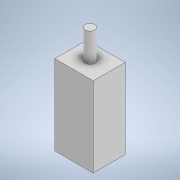
# Autodesk Inventor part: мотор_для_шестерни
Saved by Autodesk Inventor 2021.1 (Build 251245010, 245A)
## iProperties
Created: 2022-04-01
Part Number: мотор_для_шестерни
Material: Типовые
Document SubType Name: Modeling
Designer: zmoze
Density: 1 g/cm^3
Appearance: По умолчанию
Author: zmoze
Autodesk Inventor part; units mm, degrees
ref_plane "YZ Plane" through (0, 0, 0) normal (1, 0, 0) x (0, 1, 0)
ref_plane "XZ Plane" through (0, 0, 0) normal (0, 1, 0) x (-1, 0, 0)
sketch "Эскиз1" plane through (0, 0, 0) normal (0, 0, 1) x (1, 0, 0)
  line L0 (0, 0) -> (12, 0)
  line L1 (12, 0) -> (12, 25)
  line L2 (12, 25) -> (0, 25)
  line L3 (0, 25) -> (0, 0)
  dimension "d0" = 25
  dimension "d1" = 12
  constraints: 8 end point, 2 parallel, 1 horizontal, 1 perpendicular
  measures "d0" distance of L0.end L1.end
  measures "d1" distance of L1.end L2.end
extrude "Выдавливание1" add sketch "Эскиз1" along normal blind 10
sketch "Эскиз2" plane through (0, 25, 0) normal (0, 1, 0) x (1, 0, 0)
  line L0 (12, 0) -> (0, 0) construction
  line L1 (0, 0) -> (12, -10) construction
  circle A0 centre (6, -5) radius 1.5
  point P0 (12, -10)
  dimension "d4" = 3
  constraints: 2 end point, 1 centre point, 1 coincident, 1 midpoint
  measures "d4" diameter of A0
extrude "Выдавливание2" add sketch "Эскиз2" along normal blind 9
ref_plane "РабПлоскость1" through (6, 0, 0) normal (1, 0, 0) x (0, 0, -1)
